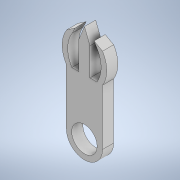
# Autodesk Inventor part: The Gripper. (New)
Saved by Autodesk Inventor 2022 (Build 260153000, 153)
## iProperties
Created: 2021-06-20
Part Number: The Gripper. (New)
Material: Generic
Document SubType Name: Modeling
Designer: fanam
Density: 1 g/cm^3
Appearance: Default
Author: fanam
Autodesk Inventor part; units mm, degrees
ref_plane "YZ Plane" through (0, 0, 0) normal (1, 0, 0) x (0, 1, 0)
ref_plane "XZ Plane" through (0, 0, 0) normal (0, 1, 0) x (-1, 0, 0)
ref_plane "XY Plane" through (0, 0, 0) normal (0, 0, 1) x (1, 0, 0)
sketch "Sketch1" plane through (0, 0, 0) normal (0, 0, 1) x (1, 0, 0)
  circle A0 centre (0, 0) radius 228.5
  arc A1 (-325, 0) -> (325, 0) centre (0, 0) ccw
  line L0 (325, 0) -> (325, 1000)
  line L1 (325, 0) -> (1325, 0) construction
  line L2 (-267.2125, -184.9932) -> (732.7875, -184.9932) construction
  line L3 (-325, 0) -> (-325, 1000)
  line L4 (-325, 0) -> (675, 0) construction
  line L5 (-225, 1000) -> (225, 1000)
  line L6 (0, 1000) -> (-100, 1000)
  line L7 (-100, 1000) -> (-100, 1500)
  line L8 (0, 1000) -> (100, 1000)
  line L9 (100, 1000) -> (100, 1500)
  arc A2 (325, 1000) -> (325, 1528.4091) centre (-99.4949, 1264.2046) ccw
  arc A3 (225, 1000) -> (225, 1526.7827) centre (-200, 1263.3913) ccw
  arc A4 (-316.0183, 1540.7518) -> (-325, 1000) centre (100, 1263.3913) ccw
  arc A5 (-216.0183, 1540.7518) -> (-225, 1000) centre (200, 1263.3913) ccw
  line L10 (-216.0183, 1540.7518) -> (-166.9198, 1640.7518)
  line L11 (-166.9198, 1640.7518) -> (-316.0183, 1540.7518)
  line L12 (225, 1526.7827) -> (173.5917, 1612.5567)
  line L13 (173.5917, 1612.5567) -> (325, 1528.4091)
  line L14 (100, 1500) -> (1.2499, 1750)
  line L15 (1.2499, 1750) -> (-100, 1500)
  point P0 (100, 1250)
  dimension "d0" = 457
  dimension "d1" = 650
  dimension "d2" = 1000
  dimension "d3" = 90
  dimension "d6" = 1000
  dimension "d7" = 90
  dimension "d8" = 100
  dimension "d9" = 500
  dimension "d10" = 100
  dimension "d11" = 500
  dimension "d12" = 500
  dimension "d13" = 200
  dimension "d14" = 500
  dimension "d15" = 300
  dimension "d16" = 100
  dimension "d17" = 500
  dimension "d18" = 500
  dimension "d19" = 100
  dimension "d20" = 200
  dimension "d22" = 100
  dimension "d23" = 100
  dimension "d25" = 300
  dimension "d26" = 100
  dimension "d27" = 30
  dimension "d28" = 30
  dimension "d29" = 100
  dimension "d30" = 250
  dimension "d31" = 43.602
  constraints: 32 end point, 11 point on circle, 6 centre point, 4 perpendicular, 4 point on line, 3 horizontal, 2 coincident, 2 midpoint, 2 tangent, 2 vertical
  measures "d0" diameter of A0
  measures "d1" diameter of A1
  measures "d2" distance of L0.start L0.end
  measures "d3" angle of L1 L0
  measures "d6" distance of L3.start L3.end
  measures "d7" angle of L4 L3
  measures "d8" distance of L6.start L6.end
  measures "d9" distance of L6.end L7.end
  measures "d10" distance of L6.start L8.end
  measures "d11" distance of L8.end L9.end
  measures "d12" radius of A2
  measures "d13" distance of point (100, 1250) A2.centre
  measures "d14" radius of A3
  measures "d15" distance from line of L9 A3.centre
  measures "d16" distance of L5.end L0.end
  measures "d17" radius of A4
  measures "d18" radius of A5
  measures "d19" distance of L5.start L3.end
  measures "d20" distance from line of L7 A4.centre
  measures "d22" distance of L11.end L10.start
  measures "d23" horizontal distance of L13.end L12.start
  measures "d25" distance from line of L7 A5.centre
  measures "d26" distance of L12.start L12.end
  measures "d27" angle of L13 L12
  measures "d28" angle of L11 L10
  measures "d29" vertical distance of L10.end L11.end
  measures "d30" vertical distance of L9.end L14.end
  measures "d31" angle of L14 L15
extrude "Extrusion1" add sketch "Sketch1" along normal blind 200
body "Solid1"
